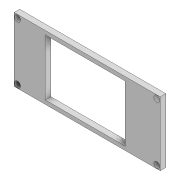
# Autodesk Inventor part: Print_Parts_TFT
Saved by Autodesk Inventor 2020.1 (Build 241239000, 239)
## iProperties
Created: 2020-11-15
Part Number: Print_Parts_TFT
Material: 一般
Document SubType Name: Modeling
Designer: kenta iguchi
Density: 1 g/cm^3
Appearance: 既定
Author: kenta iguchi
Autodesk Inventor part; units mm, degrees
ref_plane "YZ Plane" through (0, 0, 0) normal (1, 0, 0) x (0, 1, 0)
ref_plane "XZ Plane" through (0, 0, 0) normal (0, 1, 0) x (-1, 0, 0)
ref_plane "XY Plane" through (0, 0, 0) normal (0, 0, 1) x (1, 0, 0)
sketch "スケッチ1" plane through (0, 0, 0) normal (0, 0, 1) x (1, 0, 0)
  line L0 (28.75, -20.25) -> (-28.75, -20.25)
  line L1 (-28.75, -20.25) -> (-28.75, 20.25)
  line L2 (-28.75, 20.25) -> (28.75, 20.25)
  line L3 (28.75, 20.25) -> (28.75, -20.25)
  line L4 (28.75, -20.25) -> (-28.75, 20.25) construction
  line L5 (-28.75, -20.25) -> (28.75, 20.25) construction
  line L6 (-51.1, -23) -> (53.9, -23)
  line L7 (53.9, -23) -> (53.9, 23)
  line L8 (53.9, 23) -> (-51.1, 23)
  line L9 (-51.1, 23) -> (-51.1, -23)
  line L10 (-51.1, -23) -> (53.9, 23) construction
  line L11 (53.9, -23) -> (-51.1, 23) construction
  point P0 (0, 0)
  point P1 (1.4, 0)
  point P2 (1.4, 0)
  point P3 (0, 0)
  dimension "d0" = 40.5
  dimension "d1" = 57.5
  dimension "d2" = 51.1
  dimension "d4" = 53.9
  dimension "d5" = 46
  constraints: 24 end point, 6 midpoint, 4 parallel, 2 horizontal, 2 perpendicular, 1 horizontal alignment
  measures "d0" distance of L2.end L0.start
  measures "d1" distance of L0.start L0.end
  measures "d2" distance from line of point (0, 0) L9
  measures "d4" distance from line of L7 point (0, 0)
  measures "d5" distance of L6.end L7.end
extrude "押し出し1" add sketch "スケッチ1" against normal blind 4
sketch "スケッチ2" plane through (0, 0, 0) normal (0, 0, 1) x (1, 0, 0)
  line L0 (53.9, 23) -> (-51.1, 23) projected
  line L1 (-48.64, 20.575) -> (51.44, 20.575)
  line L2 (51.44, 20.575) -> (51.44, -20.575)
  line L3 (51.44, -20.575) -> (-48.64, -20.575)
  line L4 (-48.64, -20.575) -> (-48.64, 20.575)
  line L5 (-51.1, 23) -> (53.9, 23) projected
  point P0 (0, 0)
  point P1 (51.44, 0)
  point P2 (1.4, 23)
  point P3 (1.4, 20.575)
  point P4 (1.4, 23)
  dimension "d8" = 100.08
  dimension "d9" = 41.15
  constraints: 8 end point, 4 midpoint, 2 parallel, 1 horizontal, 1 horizontal alignment, 1 perpendicular, 1 vertical alignment
  measures "d8" distance of L2.end L3.end
  measures "d9" distance of L1.end L2.end
hole "穴1" at (51.44, 20.575, 0) at (51.44, -20.575, 0) at (-48.64, -20.575, 0) at (-48.64, 20.575, 0) direction (0, 0, -1) diameter 4.3 depth 8 tip angle 118
